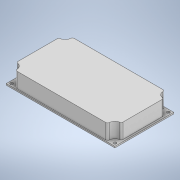
# Autodesk Inventor part: MainBoard
Saved by Autodesk Inventor 2020 (Build 240168000, 168)
## iProperties
Part Number: MainBoard
Material: 一般
Document SubType Name: Modeling
Designer: Masato Kubotera
Density: 1 g/cm^3
Appearance: 既定
Description: CircuitBoard
Author: Masato Kubotera
Autodesk Inventor part; units mm, degrees
ref_plane "YZ Plane" through (0, 0, 0) normal (1, 0, 0) x (0, 1, 0)
ref_plane "XZ Plane" through (0, 0, 0) normal (0, 1, 0) x (-1, 0, 0)
ref_plane "XY Plane" through (0, 0, 0) normal (0, 0, 1) x (1, 0, 0)
derived "Cockpit_circuit_board_frame.ipt"
sketch "スケッチ3" plane through (0, 0, -88.5) normal (0, 0, 1) x (1, 0, 0)
  line L0 (20.25, -135) -> (20.25, 0)
  line L1 (-83.25, 0) -> (-83.25, -135)
  line L2 (-31.5, -135) -> (-31.5, 0) construction
  line L3 (-83.25, -67.5) -> (20.25, -67.5) construction
  line L4 (-56.5, 1.4849) -> (-56.5, 5)
  line L5 (-56.5, 5) -> (-6.5, 5)
  line L6 (-6.5, 5) -> (-6.5, 1.4849)
  arc A0 (-57.9849, 0) -> (-56.5, 1.4849) centre (-57.2425, 0.7425) ccw
  arc A1 (-6.5, 1.4849) -> (-5.0151, 0) centre (-5.7575, 0.7425) ccw
  line L7 (-57.9849, 0) -> (-83.25, 0)
  line L8 (20.25, 0) -> (-5.0151, 0)
  line L9 (-6.5, 0) -> (-56.5, 0)
  line L10 (-6.5, -135) -> (-56.5, -135)
  arc A2 (-56.5, -136.4849) -> (-57.9849, -135) centre (-57.2425, -135.7425) ccw
  line L11 (-56.5, -136.4849) -> (-56.5, -140)
  line L12 (-56.5, -140) -> (-6.5, -140)
  line L13 (-6.5, -140) -> (-6.5, -136.4849)
  arc A3 (-5.0151, -135) -> (-6.5, -136.4849) centre (-5.7575, -135.7425) ccw
  line L14 (20.25, -135) -> (-5.0151, -135)
  line L15 (-57.9849, -135) -> (-83.25, -135)
  line L16 (18, -127.5) -> (-47, -127.5) construction
  line L17 (-47, -127.5) -> (-47, -7.5) construction
  line L18 (-47, -7.5) -> (18, -7.5) construction
  line L19 (18, -7.5) -> (18, -127.5) construction
  line L20 (18, -127.5) -> (-47, -7.5) construction
  line L21 (-47, -127.5) -> (18, -7.5) construction
  line L22 (-46, -116.5) -> (-46, -18.5)
  line L23 (-36.0627, -9.5) -> (7.0627, -9.5)
  line L24 (15, -10.5) -> (-44, -10.5) construction
  line L25 (-44, -10.5) -> (-44, -124.5) construction
  line L26 (-44, -124.5) -> (15, -124.5) construction
  line L27 (15, -124.5) -> (15, -10.5) construction
  line L28 (15, -10.5) -> (-44, -124.5) construction
  line L29 (-44, -10.5) -> (15, -124.5) construction
  circle A4 centre (15, -10.5) radius 2
  circle A5 centre (-44, -10.5) radius 2
  arc A6 (-44, -16.5) -> (-38.0471, -11.25) centre (-44, -10.5) ccw
  arc A7 (9.0471, -11.25) -> (15, -16.5) centre (15, -10.5) ccw
  line L30 (17, -18.5) -> (17, -116.5)
  line L31 (-14.5, -7.5) -> (-14.5, -127.5) construction
  line L32 (-76.25, -65) -> (-54, -65)
  line L33 (-52, -63) -> (-52, -7)
  line L34 (-54, -5) -> (-76.25, -5)
  line L35 (-78.25, -7) -> (-78.25, -63)
  arc A8 (-78.25, -63) -> (-76.25, -65) centre (-76.25, -63) ccw
  arc A9 (-54, -65) -> (-52, -63) centre (-54, -63) ccw
  arc A10 (-52, -7) -> (-54, -5) centre (-54, -7) ccw
  arc A11 (-76.25, -5) -> (-78.25, -7) centre (-76.25, -7) ccw
  arc A12 (-44, -16.5) -> (-46, -18.5) centre (-44, -18.5) ccw
  arc A13 (-36.0627, -9.5) -> (-38.0471, -11.25) centre (-36.0627, -11.5) ccw
  arc A14 (9.0471, -11.25) -> (7.0627, -9.5) centre (7.0627, -11.5) ccw
  arc A15 (17, -18.5) -> (15, -16.5) centre (15, -18.5) ccw
  line L36 (-52, -72) -> (-52, -128)
  line L37 (-78.25, -128) -> (-78.25, -72)
  arc A16 (-52, -72) -> (-54, -70) centre (-54, -72) ccw
  line L38 (-76.25, -70) -> (-54, -70)
  arc A17 (-76.25, -70) -> (-78.25, -72) centre (-76.25, -72) ccw
  line L39 (-54, -130) -> (-76.25, -130)
  arc A18 (-54, -130) -> (-52, -128) centre (-54, -128) ccw
  arc A19 (-78.25, -128) -> (-76.25, -130) centre (-76.25, -128) ccw
  arc A20 (-46, -116.5) -> (-44, -118.5) centre (-44, -116.5) ccw
  arc A21 (-38.0471, -123.75) -> (-44, -118.5) centre (-44, -124.5) ccw
  circle A22 centre (-44, -124.5) radius 2
  arc A23 (-38.0471, -123.75) -> (-36.0627, -125.5) centre (-36.0627, -123.5) ccw
  line L40 (-36.0627, -125.5) -> (7.0627, -125.5)
  arc A24 (7.0627, -125.5) -> (9.0471, -123.75) centre (7.0627, -123.5) ccw
  circle A25 centre (15, -124.5) radius 2
  arc A26 (15, -118.5) -> (9.0471, -123.75) centre (15, -124.5) ccw
  arc A27 (15, -118.5) -> (17, -116.5) centre (15, -116.5) ccw
  point P0 (0, 0)
  point P1 (-31.5, -67.5)
  point P2 (-56.5, 0)
  point P3 (-14.5, -67.5)
  point P4 (-46, -16.1569)
  point P5 (-38.0839, -9.5)
  point P6 (9.0839, -9.5)
  point P7 (17, -16.1569)
ref_plane "作業平面1" through (20.25, 0, -88.5) normal (0, 0, -1) x (0, -1, 0)
sketch "スケッチ2" plane through (20.25, 0, -88.5) normal (0, 0, -1) x (0, -1, 0)
  line L0 (127.5, 67.25) -> (7.5, 67.25) projected
  line L1 (127.5, 2.25) -> (127.5, 67.25) projected
  line L2 (7.5, 67.25) -> (7.5, 2.25) projected
  line L3 (7.5, 2.25) -> (127.5, 2.25) projected
  circle A0 centre (10.5, 64.25) radius 2 projected
  circle A1 centre (10.5, 5.25) radius 2 projected
  circle A2 centre (124.5, 64.25) radius 2 projected
  circle A3 centre (124.5, 5.25) radius 2 projected
  circle A4 centre (10.5, 5.25) radius 1.6
  circle A5 centre (10.5, 64.25) radius 1.6
  circle A6 centre (124.5, 64.25) radius 1.6
  circle A7 centre (124.5, 5.25) radius 1.6
  point P0 (0, 20.25)
  dimension "d5" = 3.2
  dimension "d6" = 3.2
  dimension "d7" = 3.2
  dimension "d8" = 3.2
  constraints: 4 centre point, 4 coincident
  measures "d5" diameter of A4
  measures "d6" diameter of A5
  measures "d7" diameter of A6
  measures "d8" diameter of A7
extrude "押し出し1" add sketch "スケッチ2" against normal blind 1.6 contours L1 L3 L2 L0 | A0 | A1 | A2 | A3
extrude "押し出し2" add sketch "スケッチ3" along normal blind 18.3 contours L22 A12 A6 A13 L23 A14 A7 A15 L30 A27 A26 A24 L40 A23 A21 A20
equation "\"d6\" = d5"
equation "\"d7\" = d5"
equation "\"d8\" = d5"
